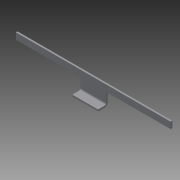
# Autodesk Inventor part: Pneumatic Puller Mount
Saved by Autodesk Inventor 2013 (Build 170138000, 138)
## iProperties
Created: 2013-02-01
Part Number: Pneumatic Puller Mount
Material: Generic
Document SubType Name: Sheet Metal
Designer: actoennies
Density: 1 g/cm^3
Sheet Metal Rule: Default
Author: actoennies
Autodesk Inventor part; units mm, degrees
ref_plane "YZ Plane" through (0, 0, 0) normal (1, 0, 0) x (0, 1, 0)
ref_plane "XZ Plane" through (0, 0, 0) normal (0, 1, 0) x (-1, 0, 0)
ref_plane "XY Plane" through (0, 0, 0) normal (0, 0, 1) x (1, 0, 0)
sketch "Sketch5" plane through (-50.8, 6.35, -3.175) normal (0, 0, 1) x (1, 0, 0)
  line L0 (0, 0) -> (50.8, 0)
  line L1 (50.8, 25.4) -> (50.8, 0)
  line L2 (50.8, 25.4) -> (101.6, 25.4)
  line L3 (101.6, 38.1) -> (-50.8, 38.1)
  line L4 (-50.8, 25.4) -> (0, 25.4)
  line L5 (0, 25.4) -> (0, 0)
  line L6 (-31.115, 23.7922) -> (-18.415, 23.7922)
  line L7 (-18.415, 20.6172) -> (-18.415, 23.7922)
  line L8 (-18.415, 20.6172) -> (-31.115, 20.6172)
  line L9 (-31.115, 20.6172) -> (-31.115, 23.7922)
  line L10 (25.4, 0) -> (25.4, 38.1) construction
  line L11 (-18.415, 20.6172) -> (-18.415, 23.7922)
  line L12 (-18.415, 23.7922) -> (-31.115, 23.7922)
  line L13 (-31.115, 23.7922) -> (-31.115, 20.6172)
  line L14 (-31.115, 20.6172) -> (-18.415, 20.6172)
  line L15 (69.215, 20.6172) -> (69.215, 23.7922)
  line L16 (69.215, 20.6172) -> (69.215, 23.7922)
  line L17 (67.6275, 25.4) -> (67.6275, 19.05)
  line L18 (67.6275, 19.05) -> (50.8, 19.05)
  line L19 (101.6, 25.4) -> (101.6, 19.05)
  line L20 (0, 19.05) -> (-16.8275, 19.05)
  line L21 (-16.8275, 19.05) -> (-16.8275, 25.4)
  line L22 (-32.7025, 25.4) -> (-32.7025, 19.05)
  line L23 (-32.7025, 19.05) -> (-50.8, 19.05)
  line L24 (-50.8, 19.05) -> (-50.8, 25.4)
  line L25 (-50.8, 38.1) -> (-50.8, 25.4)
  line L26 (69.215, 23.7922) -> (94.615, 23.7922)
  line L27 (94.615, 23.7922) -> (94.615, 20.6172)
  line L28 (94.615, 20.6172) -> (69.215, 20.6172)
  line L29 (96.2025, 25.4) -> (96.2025, 19.05)
  line L30 (96.2025, 19.05) -> (101.6, 19.05)
  point P0 (50.8, -6.35)
  point P1 (83.5025, 25.4)
  dimension "d23" = 6.35
  dimension "d25" = 1.5875
  dimension "d27" = 6.35
  dimension "d28" = 6.35
  dimension "d29" = 1.5875
  dimension "d30" = 1.5875
  dimension "d36" = 25.4
  dimension "d37" = 6.35
  dimension "d38" = 1.5875
  measures "d23" distance of L17.start L17.end
  measures "d25" distance between parallel lines of L16 L17
  measures "d27" distance between parallel lines of L4 L23
  measures "d28" distance between parallel lines of L4 L20
  measures "d29" distance between parallel lines of L7 L21
  measures "d30" distance between parallel lines of L22 L9
  measures "d36" distance of L16.end L26.end
  measures "d37" distance between parallel lines of L30 L2
  measures "d38" distance between parallel lines of L29 L27
sketch "Sketch1" plane through (0, 0, 0) normal (0, 1, 0) x (-1, 0, 0)
  line L0 (0, 0) -> (0, 12.7)
  line L1 (0, 12.7) -> (50.8, 12.7)
  line L2 (50.8, 12.7) -> (50.8, 0)
  line L3 (50.8, 0) -> (0, 0)
  dimension "d0" = 12.7
  dimension "d1" = 50.8
  measures "d0" distance of L0.start L0.end
  measures "d1" distance of L0.end L1.end
extrude "Plate1" add sketch "Sketch1" along normal blind 3.175
sketch "Sketch2" plane through (-50.8, 6.35, -3.175) normal (0, 0, -1) x (-1, 0, 0)
  line L0 (-50.8, 0) -> (0, 0)
  line L1 (0, 0) -> (0, 38.1)
  line L2 (0, 38.1) -> (-50.8, 38.1)
  line L3 (-50.8, 38.1) -> (-50.8, 0)
  constraints: 6 end point, 1 horizontal, 1 perpendicular, 1 vertical
edge flange "Flange1" height 44.45 angle 90 thickness 3.175 bend radius 3.175 thickness toward (0, 0, -1) relief straight relief width 3.175 relief depth 1.5875 edges at (-25.4, 3.175, 0) wall of the first edge with corners at (0, 6.35, -3.175) (-50.8, 6.35, -3.175) (-50.8, 44.45, -3.175) (0, 44.45, -3.175)
bend "Bend1"
corner "Corner1"
sketch "Sketch3" plane through (-50.8, 44.45, -3.175) normal (0, 0, 1) x (1, 0, 0)
  line L0 (50.8, 0) -> (50.8, -38.1)
  line L1 (0, 0) -> (0, -38.1)
  line L2 (50.8, 0) -> (101.6, 0)
  line L3 (101.6, 0) -> (101.6, -12.7)
  line L4 (101.6, -12.7) -> (50.8, -12.7)
  line L5 (0, 0) -> (-50.8, 0)
  line L6 (-50.8, 0) -> (-50.8, -12.7)
  line L7 (-50.8, -12.7) -> (0, -12.7)
  point P0 (50.8, -44.45)
  dimension "d13" = 50.8
  dimension "d14" = 12.7
  dimension "d15" = 50.8
  measures "d13" distance of L0.start L2.end
  measures "d14" distance of L2.end L3.end
  measures "d15" distance of L1.start L5.end
sheet face with bend "Face2" sketch "Sketch3" thickness 3.175 toward (0, 0, -1) bend radius 3.175 relief straight relief width 3.175 relief depth 1.5875
bend "Bend2"
sketch "Sketch4" plane through (0, 3.175, 0) normal (0, 1, 0) x (1, 0, 0)
  circle A0 centre (-43.815, -6.35) radius 3.3782 projected
  circle A1 centre (-32.7479, -6.35) radius 3.3782 projected
  circle A2 centre (-21.6807, -6.35) radius 3.3782 projected
  circle A3 centre (-10.6136, -6.35) radius 3.3782 projected
extrude "Cut1" cut sketch "Sketch4" against normal blind 3.175
sheet face with bend "Face3" sketch "Sketch5" thickness 3.175 toward (0, 0, -1) bend radius 3.175 relief straight relief width 3.175 relief depth 1.5875 contours L2 L17 L18 L1 | L2 L19 L30 L29 | L4 L22 L23 L24 | L4 L5 L20 L21
bend "Bend3"
equation "\"d21\" = Thickness"
equation "\"d3\" = BendReliefWidth"
equation "\"d4\" = BendReliefDepth"
equation "\"d5\" = MinimumRemnant"
equation "\"d6\" = BendRadius"
equation "\"d9\" = BendRadius"
equation "\"d10\" = CornerReliefSize"
equation "\"d11\" = GapSize"
equation "\"d12\" = JacobiRadiusSize"
equation "\"d16\" = BendRadius"
equation "\"d17\" = BendReliefWidth"
equation "\"d19\" = MinimumRemnant"
equation "\"d18\" = BendReliefDepth"
equation "\"d20\" = BendRadius"
equation "\"d31\" = BendRadius"
equation "\"d32\" = BendReliefWidth"
equation "\"d34\" = MinimumRemnant"
equation "\"d33\" = BendReliefDepth"
equation "\"d35\" = BendRadius"
equation "\"BendRadius\" = Thickness"
equation "\"BendReliefWidth\" = Thickness"
equation "\"BendReliefDepth\" = 0.5 * Thickness"
equation "\"CornerReliefSize\" = 4 * Thickness"
equation "\"MinimumRemnant\" = 2 * Thickness"
equation "\"TransitionRadius\" = BendRadius"
equation "\"JacobiRadiusSize\" = BendRadius"
equation "\"GapSize\" = Thickness"
equation "\"d2\" = BendRadius"
equation "\"Thickness\" = 3.175"
body "Solid1"
